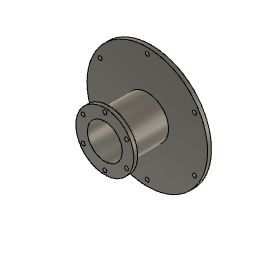
_FLANGE.3608a6b3-4ec5-4f83-87c5-ca1a5e23b2ee_LV2 (Autodesk Fusion 360 design; units mm, degrees)
Autodesk Fusion 360 part; units mm, degrees
note: some values were not read from the file. Chosen so that the rebuilt part matches the saved one: which bodies a step acts on; which pieces of a blend or face edit are solid.
sketch "Sketch1" plane through (0, 0, 0) normal (0, 1, 0) x (1, 0, 0)
  circle A0 centre (0, 0) radius 63
  circle A1 centre (0, 0) radius 78
  circle A2 centre (0, 0) radius 22.5
  circle A3 centre (0, -70.5) radius 2.5
  circle A4 centre (61.0548, -35.25) radius 2.5
  circle A5 centre (61.0548, 35.25) radius 2.5
  circle A6 centre (0, 70.5) radius 2.5
  circle A7 centre (-61.0548, 35.25) radius 2.5
  circle A8 centre (-61.0548, -35.25) radius 2.5
  dimension "d1" = 126
  dimension "d2" = 15
  dimension "d3" = 45
  dimension "d14" = 5
  dimension "d15" = 70.5
  dimension "d17" = 360
  constraint coincident A0.centre A1.centre
  constraint vertical A0.centre A3.centre
  measures "d1" diameter of A0
  measures "d2" distance of A0 A1
  measures "d3" diameter of A2
  measures "d14" diameter of A3
  measures "d15" distance of A0.centre A3.centre
extrude "Extrude1" add sketch "Sketch1" along normal blind 5 contours A1 | A3 | A4 | A5 | A6 | A7 | A8 makes body 1
move_face "OffsetFaces1" offset 65 1 faces at (62.9217, 3.3333, 3.1403) on bodies 1
extrude "Extrude2" add sketch "Sketch1" against normal blind 55 contours A2 bodies 1
sketch "Sketch3" plane through (0, -55, 0) normal (0, -1, 0) x (1, 0, 0)
  circle A0 centre (0, 0) radius 22.5
  circle A1 centre (0, 0) radius 37.5
  circle A2 centre (0, 32.5) radius 2.5
  circle A3 centre (-28.1458, 16.25) radius 2.5
  circle A4 centre (-28.1458, -16.25) radius 2.5
  circle A5 centre (0, -32.5) radius 2.5
  circle A6 centre (28.1458, -16.25) radius 2.5
  circle A7 centre (28.1458, 16.25) radius 2.5
  circle A8 centre (0, 0) radius 27.5
  dimension "d11" = 75
  dimension "d18" = 5
  dimension "d19" = 32.5
  dimension "d21" = 360
  dimension "d26" = 55
  constraint coincident A0.centre A1.centre
  constraint vertical A0.centre A2.centre
  constraint concentric A1 A8
  measures "d11" diameter of A1
  measures "d18" diameter of A2
  measures "d19" distance of A0.centre A2.centre
  measures "d26" diameter of A8
extrude "Extrude3" add sketch "Sketch3" against normal blind 5 contours A1 | A2 | A3 | A4 | A5 | A6 | A7 | A8 bodies 1
extrude "Extrude4" cut sketch "Sketch1" along normal blind 10 contours A3 | A4 | A5 | A6 | A7 | A8 bodies 1
extrude "Extrude5" cut sketch "Sketch3" against normal blind 10 contours A2 | A3 | A4 | A5 | A6 | A7 bodies 1
extrude "Extrude6" cut sketch "Sketch3" against normal blind 60 contours A0 bodies 1 makes body 2 at (-21.1632, -55, -21.5227)
extrude "Extrude7" add sketch "Sketch3" against normal blind 60 contours A8 bodies 1 2
named bodies: "Suction flange"
